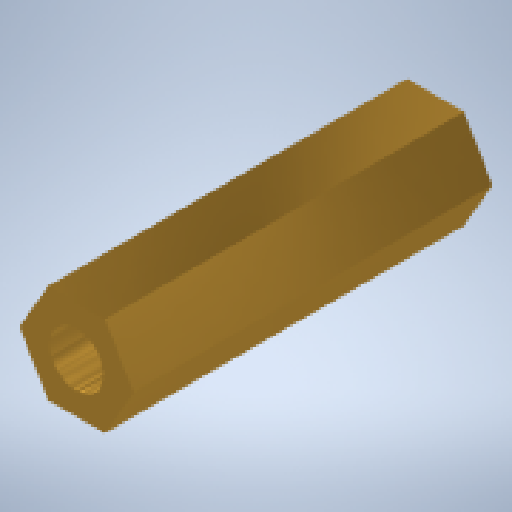
# Autodesk Inventor part: Standoff
Saved by Autodesk Inventor 2023 (Build 270158000, 158)
## iProperties
Created: 2022-08-29
Part Number: Standoff
Material: Generic
Document SubType Name: Modeling
Designer: swift
Density: 1 g/cm^3
Appearance: Brass - Satin
Author: swift
Autodesk Inventor part; units mm, degrees
ref_plane "YZ Plane" through (0, 0, 0) normal (1, 0, 0) x (0, 1, 0)
ref_plane "XZ Plane" through (0, 0, 0) normal (0, 1, 0) x (-1, 0, 0)
ref_plane "XY Plane" through (0, 0, 0) normal (0, 0, 1) x (1, 0, 0)
sketch "Sketch1" plane through (0, 0, 0) normal (0, 0, 1) x (1, 0, 0)
  arc A0 (-3.175, 3.175) -> (0, 0) centre (0.0002, 3.1752) ccw construction
  line L0 (44.45, 0) -> (0, 0) construction
  arc A1 (44.45, 0) -> (47.625, 3.175) centre (44.4498, 3.1752) ccw construction
  line L1 (47.625, 79.375) -> (47.625, 3.175) construction
  arc A2 (47.625, 79.375) -> (44.45, 82.55) centre (44.4498, 79.3748) ccw construction
  line L2 (0, 82.55) -> (44.45, 82.55) construction
  arc A3 (0, 82.55) -> (-3.175, 79.375) centre (0.0002, 79.3748) ccw construction
  line L3 (-3.175, 3.175) -> (-3.175, 79.375) construction
  circle A4 centre (0, 3.175) radius 1.6 construction
  circle A5 centre (7.112, 4.191) radius 0.51 construction
  circle A6 centre (7.112, 9.271) radius 0.51 construction
  circle A7 centre (7.112, 6.731) radius 0.51 construction
  circle A8 centre (9.652, 6.731) radius 0.51 construction
  circle A9 centre (9.652, 4.191) radius 0.51 construction
  circle A10 centre (9.652, 9.271) radius 0.51 construction
  circle A11 centre (15.655, 10.499) radius 1.15 construction
  circle A12 centre (14.225, 36.449) radius 0.85 construction
  circle A13 centre (4.699, 60.198) radius 0.51 construction
  circle A14 centre (4.699, 57.658) radius 0.51 construction
  circle A15 centre (0, 79.375) radius 1.6 construction
  circle A16 centre (4.699, 62.738) radius 0.51 construction
  circle A17 centre (4.699, 65.278) radius 0.51 construction
  circle A18 centre (13.7, 69.341) radius 0.46 construction
  circle A19 centre (16.2, 69.341) radius 0.46 construction
  circle A20 centre (6.13, 72.051) radius 1.15 construction
  circle A21 centre (11.7, 69.341) radius 0.46 construction
  circle A22 centre (9.2, 69.341) radius 0.46 construction
  circle A23 centre (23.225, 13.209) radius 0.46 construction
  circle A24 centre (25.725, 13.209) radius 0.46 construction
  circle A25 centre (18.725, 13.209) radius 0.46 construction
  circle A26 centre (21.225, 13.209) radius 0.46 construction
  circle A27 centre (28.795, 10.499) radius 1.15 construction
  circle A28 centre (44.45, 3.175) radius 1.6 construction
  circle A29 centre (30.225, 36.449) radius 0.85 construction
  circle A30 centre (39.751, 57.531) radius 0.51 construction
  circle A31 centre (39.751, 60.071) radius 0.51 construction
  circle A32 centre (31.385, 69.341) radius 0.46 construction
  circle A33 centre (33.385, 69.341) radius 0.46 construction
  circle A34 centre (19.27, 72.051) radius 1.15 construction
  circle A35 centre (28.885, 69.341) radius 0.46 construction
  circle A36 centre (25.815, 72.051) radius 1.15 construction
  circle A37 centre (39.751, 65.151) radius 0.51 construction
  circle A38 centre (39.751, 62.611) radius 0.51 construction
  circle A39 centre (35.885, 69.341) radius 0.46 construction
  circle A40 centre (38.955, 72.051) radius 1.15 construction
  circle A41 centre (44.45, 79.375) radius 1.6 construction
  circle A42 centre (0, 3.175) radius 1.5
  circle A43 centre (0, 3.175) radius 2.75 construction
  line L4 (1.5877, 0.425) -> (-1.5877, 0.425)
  line L5 (-1.5877, 0.425) -> (-3.1754, 3.175)
  line L6 (-3.1754, 3.175) -> (-1.5877, 5.925)
  line L7 (-1.5877, 5.925) -> (1.5877, 5.925)
  line L8 (1.5877, 5.925) -> (3.1754, 3.175)
  line L9 (3.1754, 3.175) -> (1.5877, 0.425)
  dimension "d0" = 3
  dimension "d1" = 5.5
  constraints: 12 end point, 3 coincident, 2 centre point, 1 horizontal, 1 tangent, 13 other
  measures "d0" diameter of A42
  measures "d1" diameter of A43
extrude "Extrusion1" add sketch "Sketch1" along normal blind 20
body "Solid1"
